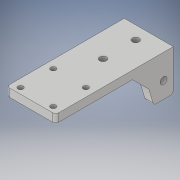
# Autodesk Inventor part: X-connector-left
Saved by Autodesk Inventor 2018 (Build 220112000, 112)
## iProperties
Created: 2017-10-12
Part Number: X-connector-left
Material: Generic
Document SubType Name: Modeling
Designer: Jurjen
Density: 1 g/cm^3
Appearance: Default
Author: Jurjen
Autodesk Inventor part; units mm, degrees
ref_plane "YZ Plane" through (0, 0, 0) normal (1, 0, 0) x (0, 1, 0)
ref_plane "XZ Plane" through (0, 0, 0) normal (0, 1, 0) x (-1, 0, 0)
ref_plane "XY Plane" through (0, 0, 0) normal (0, 0, 1) x (1, 0, 0)
sketch "Sketch1" plane through (0, 0, 0) normal (0, 1, 0) x (-1, 0, 0)
  line L0 (15, 36) -> (-15, 36)
  line L1 (-15, 36) -> (-15, -36)
  line L2 (-15, -36) -> (15, -36)
  line L3 (15, -36) -> (15, 36)
  point P0 (0, 0)
  point P1 (0, 36)
  point P2 (15, 0)
  dimension "d0" = 30
  dimension "d1" = 72
  constraints: 8 end point, 2 midpoint, 2 parallel, 1 horizontal, 1 horizontal alignment, 1 perpendicular, 1 vertical alignment
  measures "d0" distance between parallel lines of L1 L3
  measures "d1" distance between parallel lines of L0 L2
extrude "Extrusion1" add sketch "Sketch1" along normal blind 5
sketch "Sketch2" plane through (0, 5, 0) normal (0, 1, 0) x (1, 0, 0)
  circle A0 centre (-10, -12.5) radius 1.6
  circle A1 centre (-10, -32.5) radius 1.6
  circle A2 centre (10, -32.5) radius 1.6
  circle A3 centre (10, -12.5) radius 1.6
  line L0 (-10, -32.5) -> (10, -32.5) construction
  line L1 (-15, -36) -> (15, -36) projected
  point P0 (0, 0)
  point P1 (0, -32.5)
  point P2 (0, -36)
  dimension "d4" = 3.2
  dimension "d5" = 20
  dimension "d6" = 20
  dimension "d7" = 3.5
  constraints: 4 centre point, 3 equal radius, 3 vertical alignment, 2 end point, 2 horizontal alignment, 2 midpoint, 1 horizontal
  measures "d4" diameter of A1
  measures "d5" distance of L0.end L0.start
  measures "d6" distance of A0.centre L0.start
  measures "d7" distance from line of L1 L0.start
extrude "Extrusion2" cut sketch "Sketch2" against normal up to next
sketch "Sketch3" plane through (0, 5, 0) normal (0, 1, 0) x (1, 0, 0)
  line L0 (15, 36) -> (-15, 36) projected
  circle A0 centre (0, 8) radius 2.1
  circle A1 centre (0, 28) radius 2.1
  point P0 (0, 0)
  point P1 (0, 36)
  point P2 (0, 36)
  point P3 (0, 36)
  point P4 (0, 36)
  point P5 (0, 36)
  dimension "d12" = 4.2
  dimension "d14" = 20
  dimension "d52" = 8
  constraints: 5 midpoint, 5 vertical alignment, 2 centre point, 1 equal radius
  measures "d12" diameter of A1
  measures "d14" distance of A0.centre A1.centre
  measures "d52" distance from line of A1.centre L0
extrude "Extrusion3" cut sketch "Sketch3" against normal up to next
sketch "Sketch4" plane through (15, 0, 36) normal (1, 0, 0) x (0, 0, -1)
  line L0 (0, 0) -> (72, 0) projected
  line L1 (72, 0) -> (72, -20)
  line L2 (57, -10) -> (47, 0)
  line L3 (57, -10) -> (60, -20)
  line L4 (60, -20) -> (72, -20)
  line L5 (47, 0) -> (72, 0)
  point P0 (36, 0)
  point P1 (47, 5)
  point P2 (47, 5)
  point P3 (47, 5)
  dimension "d33" = 25
  dimension "d34" = 45
  dimension "d35" = 20
  dimension "d38" = 12
  constraints: 10 end point, 2 point on line, 1 collinear, 1 perpendicular, 1 vertical alignment
  measures "d33" distance of L0.end L2.end
  measures "d34" angle of L0 L2
  measures "d35" distance between parallel lines of L0 L4
  measures "d38" distance of L3.end L4.end
extrude "Extrusion4" add sketch "Sketch4" against normal blind 5
mirror "Mirror2" about plane through (0, 0, 0) normal (1, 0, 0) of "Extrusion4"
sketch "Sketch8" plane through (-15, 0, 36) normal (-1, 0, 0) x (0, 0, 1)
  circle A0 centre (-66, -10) radius 2.1
  line L0 (-60, -20) -> (-72, -20) projected
  point P0 (-36, 0)
  point P1 (-72, 0)
  point P2 (-66, -20)
  dimension "d39" = 4.2
  dimension "d40" = 10
  constraints: 1 centre point, 1 midpoint, 1 vertical alignment
  measures "d39" diameter of A0
  measures "d40" vertical distance of A0.centre point (-72, 0)
extrude "Extrusion8" cut sketch "Sketch8" against normal through all
fillet "Fillet2" radius 2 6 edges at (-12.5, -20, -36) (-12.5, -20, -24) (12.5, -20, -24) (12.5, -20, -36) (-15, 2.5, 36) (15, 2.5, 36)
sketch "Sketch9" plane through (0, 0, 0) normal (0, -1, 0) x (1, 0, 0)
  line L0 (-7, 6) -> (7, 6)
  line L1 (7, 6) -> (7, 3)
  line L2 (7, 3) -> (-7, 3)
  line L3 (-7, 3) -> (-7, 6)
  line L4 (-13, 36) -> (13, 36) projected
  point P0 (0, 0)
  point P1 (0, 3)
  dimension "d44" = 33
  dimension "d45" = 3
  dimension "d46" = 14
  constraints: 8 end point, 2 parallel, 1 horizontal, 1 midpoint, 1 perpendicular, 1 vertical alignment
  measures "d44" distance between parallel lines of L4 L2
  measures "d45" distance between parallel lines of L2 L0
  measures "d46" distance between parallel lines of L3 L1
extrude "Extrusion9" add sketch "Sketch9" along normal blind 3
chamfer "Chamfer1" distance 2 angle 45 3 edges at (-7, -3, 4.5) (0, -3, 6) (7, -3, 4.5)
ref_plane "Work Plane1" through (0, 0, 0) normal (1, 0, 0) x (0, 1, 0)
body "Solid1"
